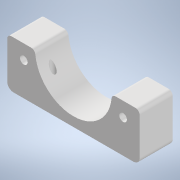
# Autodesk Inventor part: motorsupport
Saved by Autodesk Inventor 2020.1 (Build 241239000, 239)
## iProperties
Created: 2019-12-07
Part Number: motorsupport
Material: Generic
Document SubType Name: Modeling
Designer: alpha
Density: 1 g/cm^3
Appearance: Default
Author: alpha
Autodesk Inventor part; units mm, degrees
ref_plane "YZ Plane" through (0, 0, 0) normal (1, 0, 0) x (0, 1, 0)
ref_plane "XZ Plane" through (0, 0, 0) normal (0, 1, 0) x (-1, 0, 0)
ref_plane "XY Plane" through (0, 0, 0) normal (0, 0, 1) x (1, 0, 0)
sketch "Sketch1" plane through (0, 0, 0) normal (0, 0, 1) x (1, 0, 0)
  arc A0 (-18.5, 0) -> (18.5, 0) centre (0, 0) ccw projected
  line L0 (18.5, 0) -> (32.0244, 0)
  line L1 (96, -23) -> (-64, -23) projected
  circle A1 centre (24, -7) radius 1.85 projected
  circle A2 centre (-24, -7) radius 1.85 projected
  line L2 (32, -20) -> (32, 6) projected
  line L3 (-32, 6) -> (-32, -20) projected
  line L4 (-18.5, 0) -> (-32, 0)
  line L5 (-32, -20) -> (-32, -23)
  arc A3 (29, -23) -> (32, -20) centre (29, -20) ccw projected
  arc A4 (-32, -20) -> (-29, -23) centre (-29, -20) ccw projected
  point P0 (32, 0)
  constraints: 6 end point, 2 perpendicular, 2 point on line, 1 horizontal
extrude "Extrusion1" add sketch "Sketch1" along normal blind 16 contours A0 L0 L2 A3 L1 A4 L3 L4
sketch "Sketch2" plane through (-29, -23, 0) normal (0, -1, 0) x (1, 0, 0)
  circle A0 centre (45, 10) radius 1.85
  circle A1 centre (13, 10) radius 1.85
  point P0 (29, 0)
  constraints: 2 centre point, 4 other
hole "Hole1" at (16, -23, 10) at (-16, -23, 10) direction (0, 1, 0) diameter 2.7051 end through all
fillet "Fillet1" radius 2 4 edges at (32, 0, 8) (18.5, 0, 8) (-18.5, 0, 8) (-32, 0, 8)
body "Solid1"
